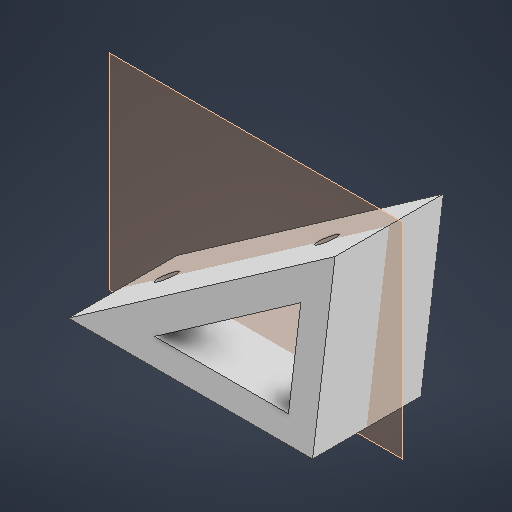
# Autodesk Inventor part: BatteryHolder
Saved by Autodesk Inventor 2026.1 (Build 301233020, 233B)
## iProperties
Created: 2025-11-11
Part Number: BatteryHolder
Material: Generic
Document SubType Name: Modeling
Designer: osama
Density: 1 g/cm^3
Appearance: Default
Author: osama
Autodesk Inventor part; units mm, degrees
ref_plane "YZ Plane" through (0, 0, 0) normal (1, 0, 0) x (0, 1, 0)
ref_plane "XZ Plane" through (0, 0, 0) normal (0, 1, 0) x (-1, 0, 0)
ref_plane "XY Plane" through (0, 0, 0) normal (0, 0, 1) x (1, 0, 0)
sketch "Sketch1" plane through (0, 0, 0) normal (0, 0, 1) x (1, 0, 0)
  line L0 (0, 0) -> (49.1491, 34.4146)
  line L1 (0, 0) -> (60, 0) construction
  line L2 (0, 0) -> (45, 0)
  line L3 (45, 0) -> (49.1491, 34.4146)
  line L4 (42.8448, 23.8964) -> (15.858, 5)
  line L5 (15.858, 5) -> (40.5666, 5)
  line L6 (40.5666, 5) -> (42.8448, 23.8964)
  dimension "d0" = 60
  dimension "d1" = 35
  dimension "d2" = 45
  dimension "d3" = 5
  constraints: 14 end point, 1 equal length, 1 horizontal, 1 point on line, 2 other
  measures "d0" distance of L0.start L0.end
  measures "d1" angle of L1 L0
  measures "d2" distance of L0.start L2.end
  measures "d3" distance between parallel lines of L0 L4
extrude "Extrusion1" add sketch "Sketch1" along normal blind 20
ref_plane "Work Plane1" through (0, 0, 10) normal (0, 0, 1) x (1, 0, 0)
sketch "Sketch2" plane through (0, 0, 0) normal (0, -1, 0) x (1, 0, 0)
  point P0 (0, 0)
  point P1 (37.6942, 10.0143)
  point P2 (8.1545, 10.0186)
hole "Hole1" at (37.6942, 0, 10.0143) at (8.1545, 0, 10.0186) direction (0, 1, 0) diameter 3.3 end through all
body "Solid1"
